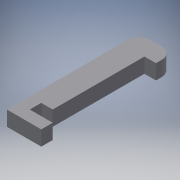
# Autodesk Inventor part: block
Saved by Autodesk Inventor 2017 (Build 210142000, 142)
## iProperties
Created: 2016-10-15
Part Number: block
Material: Generic
Document SubType Name: Modeling
Designer: Bardo91
Density: 1 g/cm^3
Appearance: Default
Author: Bardo91
Autodesk Inventor part; units mm, degrees
ref_plane "YZ Plane" through (0, 0, 0) normal (1, 0, 0) x (0, 1, 0)
ref_plane "XZ Plane" through (0, 0, 0) normal (0, 1, 0) x (-1, 0, 0)
ref_plane "XY Plane" through (0, 0, 0) normal (0, 0, 1) x (1, 0, 0)
sketch "Sketch1" plane through (0, 0, 0) normal (0, 0, 1) x (1, 0, 0)
  line L0 (0, 0) -> (-5, 0)
  line L1 (0, 0) -> (0, 5)
  line L2 (0, 5) -> (5, 5)
  line L3 (5, 5) -> (5, 45)
  line L4 (5, 45) -> (10, 45)
  line L5 (10, 45) -> (10, 47.5)
  line L6 (5, 52.5) -> (0, 52.5)
  line L7 (-5, 47.5) -> (-5, 0)
  line L8 (0, 0) -> (10, 0)
  line L9 (10, 0) -> (10, -5)
  line L10 (10, -5) -> (-5, -5)
  line L11 (-5, -5) -> (-5, 0)
  arc A0 (10, 47.5) -> (5, 52.5) centre (5, 47.5) ccw
  arc A1 (0, 52.5) -> (-5, 47.5) centre (0, 47.5) ccw
  point P0 (10, 52.5)
  point P1 (-5, 52.5)
  dimension "d0" = 5
  dimension "d1" = 5
  dimension "d2" = 5
  dimension "d3" = 40
  dimension "d4" = 5
  dimension "d5" = 7.5
  dimension "d8" = 10
  dimension "d9" = 5
  dimension "d10" = 5
  constraints: 24 end point, 8 perpendicular, 5 point on line, 4 point on circle, 4 tangent, 2 centre point, 2 vertical, 1 equal radius, 1 horizontal
  measures "d0" distance of L0.start L0.end
  measures "d1" distance of L0.start L1.end
  measures "d2" distance of L1.end L2.end
  measures "d3" distance of L2.end L3.end
  measures "d4" distance of L3.end L4.end
  measures "d5" distance of L4.end point (10, 52.5)
  measures "d8" distance of L0.start L8.end
  measures "d9" distance of L8.end L9.end
  measures "d10" radius of A0
extrude "Extrusion1" add sketch "Sketch1" along normal blind 6.5
body "Solid1"
